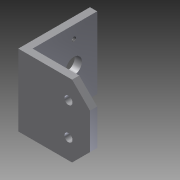
# Autodesk Inventor part: 13_0204_056
Saved by Autodesk Inventor 2012 SP1 (Build 160190100, 190)
## iProperties
Created: 2013-04-15
Part Number: 13_0204_056
Material: Default
Document SubType Name: Modeling
Designer: vogel
Density: 1 g/cm^3
Author: vogel
Autodesk Inventor part; units mm, degrees
ref_plane "YZ Plane" through (0, 0, 0) normal (1, 0, 0) x (0, 1, 0)
ref_plane "XZ Plane" through (0, 0, 0) normal (0, 1, 0) x (-1, 0, 0)
ref_plane "XY Plane" through (0, 0, 0) normal (0, 0, 1) x (1, 0, 0)
sketch "Skizze1" plane through (0, 0, 0) normal (0, 0, 1) x (1, 0, 0)
  line L0 (0, 0) -> (40, 0)
  line L1 (4, 4) -> (4, 40)
  line L2 (4, 40) -> (0, 40)
  line L3 (0, 40) -> (0, 0)
  line L4 (4, 4) -> (40, 4)
  line L5 (40, 4) -> (40, 0)
  line L6 (-8, 0) -> (48, 0) projected
  line L7 (0, -8) -> (0, 48) projected
  dimension "d0" = 40
  dimension "d3" = 40
  dimension "d4" = 4
  constraints: 12 end point, 3 perpendicular, 2 horizontal, 2 parallel
  measures "d0" distance of L2.end L0.start
  measures "d3" distance of L0.start L0.end
  measures "d4" distance of L1.end L2.end
extrude "Extrusion1" add sketch "Skizze1" along normal blind 40
sketch "Skizze2" plane through (0, 0, 0) normal (-1, 0, 0) x (0, 0, 1)
  line L0 (0, 40) -> (40, 40) projected
  line L1 (0, 0) -> (40, 0) projected
  line L2 (20, 40) -> (20, 0)
  point P0 (20, 27)
  dimension "d7" = 27
  constraints: 2 end point, 2 midpoint, 1 point on line
  measures "d7" distance from line of point (20, 27) L1
hole "Bohrung1" at (0, 27, 20) direction (1, 0, 0) diameter 9 end through all
sketch "Skizze3" plane through (0, 0, 0) normal (-1, 0, 0) x (0, 0, 1)
  circle A0 centre (20, 27) radius 4.5 projected
  line L0 (0, 40) -> (40, 40) projected
  line L1 (0, 0) -> (40, 0) projected
  line L2 (15.0773, 27) -> (4.7258, 27)
  line L3 (0, -8) -> (0, 48) projected
  line L4 (-8, 0) -> (48, 0) projected
  line L5 (20, 27) -> (20, 40)
  point P0 (7, 27)
  point P1 (33, 27)
  dimension "d15" = 13
  dimension "d16" = 26
  constraints: 4 end point, 2 point on line, 1 midpoint, 1 parallel, 1 symmetric about line
  measures "d15" distance from line of point (7, 27) L0
  measures "d16" distance of point (33, 27) point (7, 27)
hole "Bohrung2" at (0, 27, 7) at (0, 27, 33) direction (1, 0, 0) diameter 2.459 end through all thread size "M3x0.5" class "6H" standard "ISO Metric profile"
sketch "Skizze4" plane through (0, 0, 0) normal (0, -1, 0) x (1, 0, 0)
  line L0 (40, 40) -> (0, 40) projected
  line L1 (0, 0) -> (0, 40) projected
  line L2 (0, 0) -> (40, 0) projected
  line L3 (40, 0) -> (40, 40) projected
  line L4 (28, 40) -> (28, 0)
  line L5 (0, 20) -> (40, 20)
  point P0 (28, 29)
  point P1 (28, 11)
  dimension "d24" = 12
  dimension "d25" = 18
  constraints: 4 end point, 4 point on line, 2 midpoint, 1 perpendicular, 1 symmetric about line
  measures "d24" distance between parallel lines of L3 L4
  measures "d25" distance of point (28, 29) point (28, 11)
hole "Bohrung3" at (28, 0, 29) at (28, 0, 11) direction (0, 1, 0) diameter 4.5 end through all
chamfer "Fase1" distance 10 angle 45 2 edges at (40, 2, 40) (40, 2, 0)
